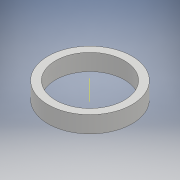
# Autodesk Inventor part: заплечик цепной передачи
Saved by Autodesk Inventor 2018.3 (Build 223284000, 284)
## iProperties
Created: 2018-05-23
Part Number: заплечик цепной передачи
Material: Типовые
Document SubType Name: Modeling
Designer: kriku
Density: 1 g/cm^3
Appearance: По умолчанию
Author: kriku
Autodesk Inventor part; units mm, degrees
ref_plane "YZ Plane" through (0, 0, 0) normal (1, 0, 0) x (0, 1, 0)
ref_plane "XZ Plane" through (0, 0, 0) normal (0, 1, 0) x (-1, 0, 0)
ref_plane "XY Plane" through (0, 0, 0) normal (0, 0, 1) x (1, 0, 0)
sketch "Эскиз1" plane through (0, 0, 0) normal (1, 0, 0) x (0, 1, 0)
  line L0 (22.5, 3.6449) -> (27.5, 3.6449)
  line L1 (27.5, 3.6449) -> (27.5, -7.2551)
  line L2 (27.5, -7.2551) -> (22.5, -7.2551)
  line L3 (22.5, -7.2551) -> (22.5, 3.6449)
  line L4 (0, -9.4351) -> (0, 5.8249) projected
  point P0 (0, 0)
  dimension "d0" = 10.9
  dimension "d1" = 22.5
  dimension "d2" = 5
  constraints: 8 end point, 3 perpendicular, 1 horizontal
  measures "d0" distance of L0.end L1.end
  measures "d1" distance from line of point (0, 0) L3
  measures "d2" distance between parallel lines of L3 L1
revolve "Вращение1" add sketch "Эскиз1" angle 360 about axis through (0, 0, -10) along (0, 0, 1)
